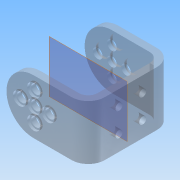
# Autodesk Inventor part: u
Saved by Autodesk Inventor 2015 (Build 190159000, 159)
## iProperties
Created: 2016-01-27
Part Number: u
Material: Plastique PMMA
Document SubType Name: Tôlerie
Designer: Gregwar
Density: 1.188 g/cm^3
Sheet Metal Rule: Par défaut_mm
Appearance: Polycarbonate - Transparent
Author: Gregwar
Autodesk Inventor part; units mm, degrees
ref_plane "YZ Plane" through (0, 0, 0) normal (1, 0, 0) x (0, 1, 0)
ref_plane "XZ Plane" through (0, 0, 0) normal (0, 1, 0) x (-1, 0, 0)
ref_plane "XY Plane" through (0, 0, 0) normal (0, 0, 1) x (1, 0, 0)
sketch "Esquisse6" plane through (20, 29, 11.5) normal (-1, 0, 0) x (0, 0, 1)
  line L0 (0, -22) -> (-23, -22) construction
  line L1 (-23, -30.3566) -> (-23, -22) construction
  line L2 (0, -30.3566) -> (-23, -30.3566) construction
  line L3 (0, -30.3566) -> (0, -22) construction
  line L4 (-23, 0) -> (0, 0) construction
  line L5 (0, 8.3566) -> (0, 0) construction
  line L6 (-23, 8.3566) -> (0, 8.3566) construction
  line L7 (-23, 8.3566) -> (-23, 0) construction
  line L8 (-23, 8.3566) -> (-23, 0) construction
  line L9 (0, 8.3566) -> (-23, 8.3566) construction
  line L10 (0, 8.3566) -> (0, 0) construction
  line L11 (0, 8.3566) -> (0, 0) construction
  line L12 (-23, -30.3566) -> (-22, -27.6783)
  line L13 (-22, -27.6783) -> (-21, -27.6783)
  line L14 (-21, -27.6783) -> (-21, -24.6783)
  line L15 (-21, -24.6783) -> (-22, -24.6783)
  line L16 (-22, -24.6783) -> (-23, -22)
  line L17 (-23, -30.3566) -> (-23, -22) construction
  line L18 (-23, -26.1783) -> (-21, -26.1783) construction
  line L19 (-23, -22) -> (-23, -30.3566)
  line L20 (-23, -30.3566) -> (0, -30.3566) projected
  line L21 (-11.5, -22) -> (-11.5, -30.3566) construction
  line L22 (-23, -22) -> (0, -22) construction
  line L23 (0, -30.3566) -> (0, -22) construction
  line L24 (-23, -30.3566) -> (0, -30.3566) construction
  line L25 (0, -30.3566) -> (-1, -27.6783)
  line L26 (-1, -27.6783) -> (-2, -27.6783)
  line L27 (-2, -27.6783) -> (-2, -24.6783)
  line L28 (-2, -24.6783) -> (-1, -24.6783)
  line L29 (-1, -24.6783) -> (0, -22)
  line L30 (0, -30.3566) -> (0, -22) construction
  line L31 (0, -26.1783) -> (-2, -26.1783) construction
  line L32 (0, -22) -> (0, -30.3566)
  line L33 (0, -30.3566) -> (-23, -30.3566)
  dimension "d31" = 1
  dimension "d32" = 1
  dimension "d33" = 3
  constraints: 48 end point, 10 symmetric about line, 4 midpoint, 3 perpendicular, 2 parallel, 1 vertical
  measures "d31" horizontal distance of L0.end L15.end
  measures "d32" distance of L14.end L15.end
  measures "d33" distance between parallel lines of L13 L15
sketch "Esquisse1" plane through (0, 0, 0) normal (0, 1, 0) x (-1, 0, 0)
  arc A0 (0, -11.5) -> (0, 11.5) centre (0, 0) ccw
  line L0 (0, 11.5) -> (-20, 11.5)
  line L1 (-20, 11.5) -> (-20, -11.5)
  line L2 (-20, -11.5) -> (0, -11.5)
  dimension "d0" = 23
  dimension "d1" = 20
  dimension "d2" = 11.5
  measures "d0" distance between parallel lines of L0 L2
  measures "d1" distance from line of point (0, 0) L1
  measures "d2" radius of A0
extrude "Plaque1" add sketch "Esquisse1" along normal blind 3
sketch "Esquisse2" plane through (0, 0, 0) normal (0, -1, 0) x (1, 0, 0)
  arc A0 (0, 11.5) -> (0, -11.5) centre (0, 0) ccw construction
  line L0 (0, 0) -> (-6, 0) construction
  point P0 (0, 6)
  point P1 (0, -6)
  point P2 (6, 0)
  dimension "d6" = 360
  dimension "d8" = 6
  constraints: 3 coincident, 2 end point, 1 horizontal, 5 other
  measures "d8" distance of point (0, 0) point (0, 6)
hole "Perçage1" at (0, 0, 0) at (0, 0, 6) at (-6, 0, 0) at (0, 0, -6) at (6, 0, 0) direction (0, 1, 0) diameter 4.05 end through all counterbore diameter 5.5 counterbore depth 1
ref_plane "Plan de construction1" through (0, 18, 0) normal (0, 1, 0) x (1, 0, 0)
mirror "Symétrie1" about plane through (0, 18, 0) normal (0, 1, 0)
sketch "Esquisse3" plane through (20, 0, 11.5) normal (1, 0, 0) x (0, 0, -1)
  line L0 (23, 3) -> (0, 3)
  line L1 (0, 0) -> (0, 3)
  line L2 (23, 0) -> (0, 0)
  line L3 (23, 0) -> (23, 3)
  line L4 (23, 33) -> (0, 33)
  line L5 (23, 36) -> (23, 33)
  line L6 (23, 36) -> (0, 36)
  line L7 (0, 36) -> (0, 33)
  line L8 (0, 0) -> (23, 0)
  line L9 (23, 0) -> (23, 36)
  line L10 (23, 36) -> (0, 36)
  line L11 (0, 36) -> (0, 0)
  point P0 (11.5, 0)
sheet face with bend "Face2" sketch "Esquisse3" thickness 3 toward (1, 0, 0) bend radius 4 contours L0 L11 L4 L9
bend "Pli1"
sketch "Esquisse4" plane through (23, 0, 11.5) normal (1, 0, 0) x (0, 0, -1)
  line L0 (23, 7) -> (0, 7) construction
  line L1 (23, 29) -> (23, 7) construction
  line L2 (0, 29) -> (23, 29) construction
  line L3 (0, 7) -> (0, 29) construction
  line L4 (23, 18) -> (0, 18) construction
  circle A0 centre (16.5, 23) radius 1.5
  line L5 (11.5, 18) -> (11.5, 7) construction
  circle A1 centre (16.5, 13) radius 1.5
  circle A2 centre (6.5, 23) radius 1.5
  circle A3 centre (6.5, 13) radius 1.5
  point P0 (11.5, 0)
  dimension "d22" = 10
  dimension "d23" = 3
  dimension "d25" = 10
  constraints: 4 centre point, 4 end point, 4 midpoint, 3 symmetric about line, 3 other
  measures "d22" distance of A0.centre A1.centre
  measures "d23" diameter of A0
  measures "d25" distance of A2.centre A0.centre
extrude "Couper1" cut sketch "Esquisse4" against normal blind 3
equation "\"d8\" = ollo_spacing"
equation "\"d2\" = 0.5 * d0"
equation "\"d9\" = ollo_hole"
equation "\"d11\" = ollo_ring"
equation "\"d12\" = ollo_depth"
equation "\"d14\" = Epaisseur"
equation "\"d25\" = d22"
equation "\"d26\" = Epaisseur"
equation "\"d17\" = RayonPli"
equation "\"d18\" = LargeurGrugeage"
equation "\"d20\" = RestesMinimum"
equation "\"d19\" = ProfondeurGrugeage"
equation "\"d21\" = RayonPli"
equation "\"LargeurGrugeage\" = Epaisseur"
equation "\"ProfondeurGrugeage\" = 0.5 * Epaisseur"
equation "\"TailleGrugeage\" = 4 * Epaisseur"
equation "\"RestesMinimum\" = 2 * Epaisseur"
equation "\"Rayondetransition\" = RayonPli"
equation "\"TailleRayonJacobi\" = RayonPli"
equation "\"TailleJeu\" = Epaisseur"
equation "\"d3\" = RayonPli"
equation "\"ollo_hole\" = 4.05"
equation "\"ollo_ring\" = 5.5"
equation "\"ollo_depth\" = 1"
equation "\"Epaisseur\" = 3"
equation "\"RayonPli\" = 4"
equation "\"ollo_spacing\" = 6"
